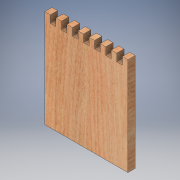
# Autodesk Inventor part: cabinet-side
Saved by Autodesk Inventor 2016 (Build 200138000, 138)
## iProperties
Created: 2015-10-24
Part Number: cabinet-side
Material: Wood (Birch)
Document SubType Name: Modeling
Designer: jeremyhale
Density: 0.55 g/cm^3
Appearance: Birch - Natural Polished
Mass: 530.129 g
Surface Area: 1289.44 cm^2
Volume: 963.87 cm^3
Author: jeremyhale
Autodesk Inventor part; units mm, degrees
ref_plane "YZ Plane" through (0, 0, 0) normal (1, 0, 0) x (0, 1, 0)
ref_plane "XZ Plane" through (0, 0, 0) normal (0, 1, 0) x (-1, 0, 0)
ref_plane "XY Plane" through (0, 0, 0) normal (0, 0, 1) x (1, 0, 0)
sketch "Sketch4" plane through (0, 0, 0) normal (0, 0, 1) x (1, 0, 0)
  line L0 (-107.95, -127) -> (107.95, -127)
  line L1 (107.95, -127) -> (107.95, 127)
  line L2 (107.95, 127) -> (-107.95, 127)
  line L3 (-107.95, 127) -> (-107.95, -127)
  line L4 (-107.95, -127) -> (107.95, 127) construction
  line L5 (107.95, -127) -> (-107.95, 127) construction
  point P0 (0, 0)
  dimension "width" = 215.9
  dimension "height" = 254
  constraints: 12 end point, 2 midpoint, 2 parallel, 1 horizontal, 1 perpendicular
  measures "width" distance of L1.end L2.end
  measures "height" distance of L0.end L1.end
extrude "Extrusion3" add sketch "Sketch4" along normal blind 19
sketch "Sketch6" plane through (0, 0, 19) normal (0, 0, 1) x (1, 0, 0)
  line L0 (107.95, -127) -> (107.95, 127) projected
  line L1 (-107.95, 127) -> (-107.95, -127) projected
  line L2 (107.95, 127) -> (-107.95, 127) projected
  line L3 (-107.95, 127) -> (-93.5567, 127) construction
  line L4 (-93.5567, 127) -> (-93.5567, 108)
  line L5 (-93.5567, 108) -> (-79.1633, 108)
  line L6 (-79.1633, 108) -> (-79.1633, 127)
  line L7 (-79.1633, 127) -> (-93.5567, 127)
  point P0 (0, 0)
  dimension "d37" = 215.9
  dimension "d38" = 14.3933
  dimension "d39" = 19
  dimension "d40" = 14.3933
  dimension "d41" = 19
  constraints: 10 end point, 2 perpendicular, 2 point on line
  measures "d37" distance between parallel lines of L0 L1
  measures "d38" distance of L1.start L3.end
  measures "d39" distance of L3.end L4.end
  measures "d40" distance of L4.end L5.end
  measures "d41" distance of L5.end L6.end
extrude "Extrusion4" cut sketch "Sketch6" against normal blind 19
pattern_linear "Rectangular Pattern1" count 7 spacing 28.7867 along (1, 0, 0) of "Extrusion4"
sketch "Sketch9" plane through (0, 0, 0) normal (0, 0, -1) x (-1, 0, 0)
  point P0 (-50.8, -76.5625)
hole "Hole3" at (50.8, -76.5625, 0) direction (0, 0, 1) diameter 6.6 depth 19 countersink diameter 12.6 countersink angle 90
sketch "Sketch10" plane through (0, 0, 0) normal (0, 0, -1) x (-1, 0, 0)
  point P0 (50.8, -76.5625)
hole "Hole4" at (-50.8, -76.5625, 0) direction (0, 0, 1) diameter 6.6 depth 19 countersink diameter 12.6 countersink angle 90
equation "\"d24\" = thickness"
equation "\"d39\" = thickness"
equation "\"d41\" = thickness"
equation "\"d42\" = thickness"
equation "\"thickness\" = 19"
body "Solid1"
